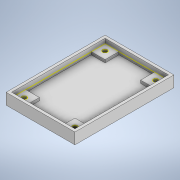
# Autodesk Inventor part: PCB_REMOTE_Holder_
Saved by Autodesk Inventor 2021 (Build 250183000, 183)
## iProperties
Created: 2021-04-21
Part Number: PCB_REMOTE_Holder_
Material: Generic
Document SubType Name: Modeling
Designer: Patrick
Density: 1 g/cm^3
Appearance: Default
Author: Patrick
Autodesk Inventor part; units mm, degrees
ref_plane "YZ Plane" through (0, 0, 0) normal (1, 0, 0) x (0, 1, 0)
ref_plane "XZ Plane" through (0, 0, 0) normal (0, 1, 0) x (-1, 0, 0)
ref_plane "XY Plane" through (0, 0, 0) normal (0, 0, 1) x (1, 0, 0)
sketch "Sketch1" plane through (0, 0, 0) normal (0, 1, 0) x (-1, 0, 0)
  line L0 (0, 0) -> (50.175, 0)
  line L1 (50.175, 0) -> (50.175, -77.485)
  line L2 (50.175, -77.485) -> (0, -77.485)
  line L3 (0, -77.485) -> (0, 0)
  circle A0 centre (48.265, -1.91) radius 2.1
  circle A1 centre (48.265, -75.575) radius 2.1
  circle A2 centre (1.91, -1.91) radius 2.1
  circle A3 centre (1.91, -75.575) radius 2.1
  line L4 (50.175, 0) -> (53.985, 0)
  line L5 (53.985, 0) -> (53.985, -77.675)
  line L6 (53.985, -77.675) -> (50.175, -77.675)
  line L7 (50.175, -77.675) -> (50.175, 0)
  line L8 (0, 0) -> (-3.81, 0)
  line L9 (-3.81, 0) -> (-3.81, -77.675)
  line L10 (-3.81, -77.675) -> (0, -77.675)
  line L11 (0, -77.675) -> (0, 0)
  line L12 (53.985, -77.675) -> (-3.81, -77.675)
  line L13 (-3.81, -77.675) -> (-3.81, -81.485)
  line L14 (-3.81, -81.485) -> (53.985, -81.485)
  line L15 (53.985, -81.485) -> (53.985, -77.675)
  line L16 (-3.81, 0) -> (53.985, 0)
  line L17 (53.985, 0) -> (53.985, 3.81)
  line L18 (53.985, 3.81) -> (-3.81, 3.81)
  line L19 (-3.81, 3.81) -> (-3.81, 0)
  point P0 (0, -77.485)
  point P1 (0, -76.4479)
  point P2 (0, -74.7021)
  point P3 (0, -2.7829)
  point P4 (0, -1.0371)
  dimension "d0" = 77.485
  dimension "d1" = 50.175
  dimension "d3" = 4.2
  dimension "d4" = 4.2
  dimension "d6" = 1.91
  dimension "d7" = 1.91
  dimension "d8" = 1.91
  dimension "d9" = 4.2
  dimension "d10" = 4.2
  dimension "d11" = 1.91
  dimension "d12" = 1.91
  dimension "d13" = 1.91
  dimension "d14" = 1.91
  dimension "d15" = 1.91
  dimension "d18" = 3.81
  dimension "d19" = 3.81
  dimension "d20" = 3.81
  dimension "d21" = 3.81
  constraints: 40 end point, 10 parallel, 5 horizontal, 5 perpendicular, 4 centre point, 1 point on line
  measures "d0" distance of L2.end L0.start
  measures "d1" distance between parallel lines of L3 L1
  measures "d3" diameter of A1
  measures "d4" diameter of A0
  measures "d6" distance from line of L1 A0.centre
  measures "d7" distance from line of L2 A1.centre
  measures "d8" distance from line of A0.centre L0
  measures "d9" diameter of A2
  measures "d10" diameter of A3
  measures "d11" distance from line of L0 A2.centre
  measures "d12" distance from line of A2.centre L3
  measures "d13" distance from line of L2 A3.centre
  measures "d14" distance from line of L3 A3.centre
  measures "d15" distance from line of L1 A1.centre
  measures "d18" distance of L5.end L6.end
  measures "d19" distance of L10.end L9.end
  measures "d20" distance of L13.end L12.end
  measures "d21" distance of L17.end L16.end
extrude "Extrusion2" add sketch "Sketch1" along normal blind 6 contours L8 L19 L18 L17 L4 L0 A0 A2 | L0 A2 L3 | L3 A2 A3 L11 L10 L9 L8 | L0 A0 L1 A1 L2 A3 L3 A2 | L10 L12 L6 L15 L14 L13 | L11 L2 A3 L12 | L0 L1 A0 | A0 L1 L4 L5 L6 L7 A1 | A3 L2 L3 | A3 L2 A1 L12 | A1 L2 L7 L12 | L1 L2 A1 picked at (0.2904, -0.2904) picked at (49.8846, -0.2904) picked at (0.2904, -77.1946) picked at (49.8846, -77.1946)
sketch "Sketch2" plane through (0, 6, 0) normal (0, 1, 0) x (1, 0, 0)
  circle A0 centre (-1.91, 1.91) radius 2.1 projected
  circle A1 centre (-48.265, 1.91) radius 2.1 projected
  circle A2 centre (-48.265, 75.575) radius 2.1 projected
  line L0 (3.81, -3.81) -> (3.81, 81.485) projected
  line L1 (3.81, 81.485) -> (-53.985, 81.485) projected
  line L2 (-53.985, 81.485) -> (-53.985, -3.81) projected
  line L3 (-53.985, -3.81) -> (3.81, -3.81) projected
  circle A3 centre (-1.91, 75.575) radius 2.1 projected
  point P0 (0, 0)
sketch "Sketch3" plane through (0, 0, 0) normal (0, -1, 0) x (1, 0, 0)
  line L0 (-53.985, 3.81) -> (3.81, 3.81) projected
  line L1 (-53.985, 3.81) -> (3.81, 3.81)
  line L2 (3.81, 3.81) -> (3.81, 6.35)
  line L3 (3.81, 6.35) -> (-53.985, 6.35)
  line L4 (-53.985, 6.35) -> (-53.985, 3.81)
  circle A0 centre (-1.91, -1.91) radius 2.1 projected
  circle A1 centre (-48.265, -1.91) radius 2.1 projected
  circle A2 centre (-48.265, -75.575) radius 2.1 projected
  line L5 (3.81, 3.81) -> (3.81, -81.485) projected
  line L6 (-53.985, 3.81) -> (3.81, 3.81) projected
  line L7 (-53.985, -81.485) -> (-53.985, 3.81) projected
  line L8 (3.81, -81.485) -> (-53.985, -81.485) projected
  circle A3 centre (-1.91, -75.575) radius 2.1 projected
  line L9 (3.81, 6.35) -> (6.35, 6.35)
  line L10 (6.35, 6.35) -> (6.35, -81.485)
  line L11 (6.35, -81.485) -> (3.81, -81.485)
  line L12 (3.81, -81.485) -> (3.81, 6.35)
  line L13 (3.81, -81.485) -> (-53.985, -81.485) projected
  line L14 (-53.985, -81.485) -> (6.35, -81.485)
  line L15 (6.35, -81.485) -> (6.35, -84.025)
  line L16 (6.35, -84.025) -> (-53.985, -84.025)
  line L17 (-53.985, -84.025) -> (-53.985, -81.485)
  line L18 (-53.985, 6.35) -> (-56.525, 6.35)
  line L19 (-56.525, 6.35) -> (-56.525, -84.025)
  line L20 (-56.525, -84.025) -> (-53.985, -84.025)
  line L21 (-53.985, -84.025) -> (-53.985, 6.35)
  point P0 (0, 0)
  dimension "d24" = 2.54
  dimension "d25" = 2.54
  dimension "d26" = 2.54
  dimension "d27" = 2.54
  constraints: 32 end point, 8 parallel, 4 horizontal, 4 perpendicular, 2 point on line
  measures "d24" distance of L2.end L1.end
  measures "d25" distance of L10.end L11.end
  measures "d26" distance of L14.end L15.end
  measures "d27" distance of L20.end L19.end
extrude "Extrusion3" add sketch "Sketch3" against normal blind 10.16 contours L4 L3 L2 L0 | L7 L17 L20 L19 L18 L4 | L2 L9 L10 L11 L5 | L8 L11 L15 L16 L17
sketch "Sketch4" plane through (0, 6, 0) normal (0, 1, 0) x (1, 0, 0)
  point P0 (0, 0)
sketch "Sketch5" plane through (0, 6, 0) normal (0, 1, 0) x (1, 0, 0)
  circle A0 centre (-1.91, 1.91) radius 2.1 projected
  circle A1 centre (-48.265, 1.91) radius 2.1 projected
  circle A2 centre (-48.265, 75.575) radius 2.1 projected
  line L0 (3.81, -3.81) -> (3.81, 81.485) projected
  line L1 (3.81, 81.485) -> (-53.985, 81.485) projected
  line L2 (-53.985, 81.485) -> (-53.985, -3.81) projected
  line L3 (-53.985, -3.81) -> (3.81, -3.81) projected
  circle A3 centre (-1.91, 75.575) radius 2.1 projected
  line L4 (-56.525, 84.025) -> (-56.525, -6.35) projected
  line L5 (-53.985, -3.81) -> (-53.985, 81.485) projected
  line L6 (-53.985, -3.81) -> (3.81, 81.485)
  line L7 (-53.985, 81.485) -> (-53.985, -3.81) projected
  line L8 (-53.985, 81.485) -> (3.81, -3.81)
  line L9 (-53.985, 81.485) -> (-41.285, 81.485)
  line L10 (-41.285, 81.485) -> (-41.285, 68.785)
  line L11 (-41.285, 68.785) -> (-53.985, 68.785)
  line L12 (-53.985, 68.785) -> (-53.985, 81.485)
  line L13 (3.81, 81.485) -> (-53.985, 81.485) projected
  line L14 (3.81, 81.485) -> (-8.89, 81.485)
  line L15 (-8.89, 81.485) -> (-8.89, 68.785)
  line L16 (-8.89, 68.785) -> (3.81, 68.785)
  line L17 (3.81, 68.785) -> (3.81, 81.485)
  line L18 (-53.985, -3.81) -> (3.81, -3.81) projected
  line L19 (-53.985, -3.81) -> (-41.285, -3.81)
  line L20 (-41.285, -3.81) -> (-41.285, 8.89)
  line L21 (-41.285, 8.89) -> (-53.985, 8.89)
  line L22 (-53.985, 8.89) -> (-53.985, -3.81)
  line L23 (3.81, -3.81) -> (-8.89, -3.81)
  line L24 (-8.89, -3.81) -> (-8.89, 8.89)
  line L25 (-8.89, 8.89) -> (3.81, 8.89)
  line L26 (3.81, 8.89) -> (3.81, -3.81)
  point P0 (0, 0)
  dimension "d30" = 12.7
  dimension "d31" = 12.7
  dimension "d32" = 12.7
  dimension "d33" = 12.7
  dimension "d34" = 12.7
  dimension "d35" = 12.7
  constraints: 36 end point, 8 parallel, 4 horizontal, 4 perpendicular, 1 point on line
  measures "d30" distance of L10.end L11.end
  measures "d31" distance of L9.end L10.end
  measures "d32" distance of L16.end L15.end
  measures "d33" distance of L15.end L14.end
  measures "d34" distance of L21.end L20.end
  measures "d35" distance of L20.end L19.end
extrude "Extrusion4" cut sketch "Sketch5" against normal blind 2.54 contours L25 L24 L3 L20 L21 L6 L8 | L8 L6 L16 L0 L25 | L8 L11 L10 L1 L15 L16 L6 | L6 L21 L2 L11 L8
body "Solid2"
